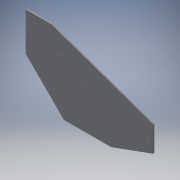
# Autodesk Inventor part: endplate
Saved by Autodesk Inventor 2018.2 (Build 222227000, 227)
## iProperties
Created: 2018-02-23
Part Number: endplate
Material: 一般
Document SubType Name: Modeling
Designer: ku_sk
Density: 1 g/cm^3
Appearance: 既定
Author: ku_sk
Autodesk Inventor part; units mm, degrees
ref_plane "YZ Plane" through (0, 0, 0) normal (1, 0, 0) x (0, 1, 0)
ref_plane "XZ Plane" through (0, 0, 0) normal (0, 1, 0) x (-1, 0, 0)
ref_plane "XY Plane" through (0, 0, 0) normal (0, 0, 1) x (1, 0, 0)
sketch "スケッチ1" plane through (0, 0, 0) normal (0, 1, 0) x (-1, 0, 0)
  line L0 (-277.5, 280) -> (277.5, 280)
  line L1 (277.5, 280) -> (277.5, -280)
  line L2 (277.5, -280) -> (-277.5, -280)
  line L3 (-277.5, -280) -> (-277.5, 280)
  line L4 (-277.5, 280) -> (277.5, -280) construction
  line L5 (277.5, 280) -> (-277.5, -280) construction
  point P0 (0, 0)
  dimension "d0" = 555
  dimension "d1" = 560
  constraints: 12 end point, 2 midpoint, 2 parallel, 1 horizontal, 1 perpendicular
  measures "d0" distance of L0.start L0.end
  measures "d1" distance of L2.end L0.start
extrude "押し出し1" add sketch "スケッチ1" along normal mid plane 5
sketch "スケッチ3" plane through (0, -2.5, 0) normal (0, -1, 0) x (1, 0, 0)
  circle A0 centre (-62.5, 115) radius 2.5
  line L0 (277.5, -280) -> (277.5, 280) projected
  line L1 (-277.5, -280) -> (277.5, -280) projected
  circle A1 centre (-162.5, 190) radius 2.5
  circle A2 centre (257.5, 40) radius 2.5
  point P0 (0, 0)
  dimension "d10" = 5
  dimension "d15" = 5
  dimension "d16" = 320
  dimension "d17" = 20
  dimension "d18" = 5
  dimension "d24" = 75
  dimension "d25" = 320
  dimension "d26" = 420
  dimension "d27" = 150
  constraints: 3 centre point
  measures "d10" diameter of A0
  measures "d15" diameter of A1
  measures "d16" distance from line of L1 A2.centre
  measures "d17" distance from line of L0 A2.centre
  measures "d18" diameter of A2
  measures "d24" vertical distance of A0.centre A2.centre
  measures "d25" horizontal distance of A0.centre A2.centre
  measures "d26" horizontal distance of A1.centre A2.centre
  measures "d27" vertical distance of A2.centre A1.centre
extrude "押し出し4" cut sketch "スケッチ3" against normal through all
sketch "スケッチ5" plane through (0, -2.5, 0) normal (0, -1, 0) x (1, 0, 0)
  line L0 (277.5, 250) -> (-277.5, 250)
  line L1 (-250, 280) -> (-250, -280) construction
  line L2 (-277.5, -250) -> (277.5, -250)
  line L3 (250, -280) -> (250, 280) construction
  line L4 (-277.5, 280) -> (277.5, 280)
  line L5 (-150, 280) -> (277.5, 120)
  line L6 (277.5, 280) -> (277.5, -280)
  line L7 (-277.5, -280) -> (-277.5, 280)
  line L8 (-277.5, 120) -> (-150.482941, -100)
  line L9 (-150.482941, -100) -> (277.5, -100)
  line L10 (277.5, -280) -> (277.5, 280)
  point P0 (0, 0)
  dimension "d32" = 100
  dimension "d33" = 130
  dimension "d34" = 350
  dimension "d35" = 60
  dimension "d46" = 220
  constraints: 6 end point, 4 point on line, 1 horizontal, 1 vertical alignment
  measures "d32" distance from line of L5.start L1
  measures "d33" distance from line of L0 L8.start
  measures "d34" distance between parallel lines of L0 L9
  measures "d35" angle of L9 L8
  measures "d46" distance of L9.end L5.end
sketch "スケッチ5 outline for 押し出し5" plane through (0, -2.5, 0) normal (0, -1, 0) x (1, 0, 0)
  line L0 (277.5, 120) -> (277.5, 280)
  line L1 (-150, 280) -> (277.5, 120)
  line L2 (277.5, 280) -> (-150, 280)
  line L3 (-277.5, 120) -> (-277.5, -280)
  line L4 (-150.482941, -100) -> (-277.5, 120)
  line L5 (277.5, -100) -> (-150.482941, -100)
  line L6 (277.5, -280) -> (277.5, -100)
  line L7 (-277.5, -280) -> (277.5, -280)
extrude "押し出し5" cut sketch "スケッチ5 outline for 押し出し5" against normal through all
chamfer "面取り2" distance 170 distance2 100 1 edges at (-150.4829, 0, -100) measured on face at (134.839, -0.8333, -100)
